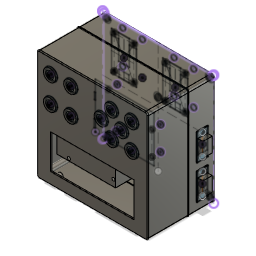
ArduinoController v4 (Autodesk Fusion 360 design; units mm, degrees)
Autodesk Fusion 360 part; units mm, degrees
sketch "Sketch1" plane through (0, 0, 0) normal (0, 0, 1) x (1, 0, 0) in component "RelayBoard"
  line L0 (22.5, -14.5) -> (-22.5, -14.5)
  line L1 (-22.5, -14.5) -> (-22.5, 14.5)
  line L2 (-22.5, 14.5) -> (22.5, 14.5)
  line L3 (22.5, 14.5) -> (22.5, -14.5)
  line L4 (22.5, -14.5) -> (-22.5, 14.5) construction
  line L5 (-22.5, -14.5) -> (22.5, 14.5) construction
  line L6 (19.5, -11.5) -> (-19.5, -11.5) construction
  line L7 (-19.5, -11.5) -> (-19.5, 11.5) construction
  line L8 (-19.5, 11.5) -> (19.5, 11.5) construction
  line L9 (19.5, 11.5) -> (19.5, -11.5) construction
  line L10 (19.5, -11.5) -> (-19.5, 11.5) construction
  line L11 (-19.5, -11.5) -> (19.5, 11.5) construction
  circle A0 centre (-19.5, 11.5) radius 1.75
  circle A1 centre (-19.5, 11.5) radius 1
  line L12 (0, 14.5) -> (0, -14.5) construction
  line L13 (-22.5, 0) -> (22.5, 0) construction
  circle A2 centre (19.5, 11.5) radius 1
  circle A3 centre (19.5, 11.5) radius 1.75
  circle A4 centre (19.5, -11.5) radius 1.75
  circle A5 centre (19.5, -11.5) radius 1
  circle A6 centre (-19.5, -11.5) radius 1
  circle A7 centre (-19.5, -11.5) radius 1.75
  line L14 (-22.5, 5.75) -> (-14.5, 5.75)
  line L15 (-14.5, 5.75) -> (-14.5, -5.75)
  line L16 (-14.5, -5.75) -> (-22.5, -5.75)
  line L17 (-22.5, -5.75) -> (-22.5, 5.75)
  line L18 (-22.5, 0) -> (-14.5, 0) construction
  line L19 (22.5, 6.15) -> (-6.5, 6.15)
  line L20 (-6.5, 6.15) -> (-6.5, -6.15)
  line L21 (-6.5, -6.15) -> (22.5, -6.15)
  line L22 (22.5, -6.15) -> (22.5, 6.15)
  line L23 (-6.5, 0) -> (22.5, 0) construction
  line L24 (16.1, 14.5) -> (4.6, 14.5)
  line L25 (4.6, 14.5) -> (4.6, 6.5)
  line L26 (4.6, 6.5) -> (16.1, 6.5)
  line L27 (16.1, 6.5) -> (16.1, 14.5)
  line L28 (4.6, -14.5) -> (4.6, -6.5)
  line L29 (4.6, -6.5) -> (16.1, -6.5)
  line L30 (16.1, -14.5) -> (4.6, -14.5)
  line L31 (16.1, -6.5) -> (16.1, -14.5)
  dimension "d1" = 45
  dimension "d2" = 29
  dimension "d3" = 39
  dimension "d4" = 23
  dimension "d5" = 3.5
  dimension "d6" = 2
  dimension "d7" = 11.5
  dimension "d8" = 29
  dimension "d9" = 12.3
  dimension "d10" = 8
  dimension "d11" = 11.5
  dimension "d12" = 8
  dimension "d13" = 6.4
  constraint horizontal L0
  constraint perpendicular L0 L1
  constraint parallel L0 L2
  constraint parallel L1 L3
  constraint coincident L4 origin
  constraint coincident L5 origin
  constraint horizontal L6
  constraint perpendicular L6 L7
  constraint parallel L6 L8
  constraint parallel L7 L9
  constraint coincident L10 origin
  constraint coincident L11 origin
  constraint coincident L7.end L8.start
  constraint concentric A0 A1
  constraint midpoint L2 L12.start
  constraint midpoint L0 L12.end
  constraint midpoint L1 L13.start
  constraint midpoint L3 L13.end
  constraint symmetric A0 L12 A3
  constraint symmetric A1 L12 A2
  constraint symmetric A0 L13 A7
  constraint symmetric A1 L13 A6
  constraint symmetric L13 A2 A5
  constraint symmetric L13 A3 A4
  constraint horizontal L14
  constraint vertical L15
  constraint horizontal L16
  constraint vertical L17
  constraint coincident L1 L14.start
  constraint midpoint L17 L13.start
  constraint midpoint L15 L18.end
  constraint collinear L13 L18
  constraint horizontal L19
  constraint vertical L20
  constraint horizontal L21
  constraint vertical L22
  constraint coincident L3 L19.start
  constraint midpoint L20 L23.start
  constraint midpoint L22 L13.end
  constraint collinear L13 L23
  constraint horizontal L24
  constraint vertical L25
  constraint horizontal L26
  constraint vertical L27
  constraint coincident L2 L24.start
  constraint symmetric L13 L24.start L30.start
  constraint symmetric L13 L24.end L28.start
  constraint symmetric L13 L25.end L28.end
  constraint symmetric L13 L26.end L29.end
  measures "d1" distance of L1.end L2.end
  measures "d2" distance of L0.end L1.end
  measures "d3" distance of L7.end L8.end
  measures "d4" distance of L6.end L7.end
  measures "d5" diameter of A0
  measures "d6" diameter of A1
  measures "d7" distance of L14.start L16.end
  measures "d8" distance of L19.start L19.end
  measures "d9" distance of L19.start L21.end
  measures "d10" distance of L15.end L16.end
  measures "d11" distance of L24.start L24.end
  measures "d12" distance of L24.start L26.end
  measures "d13" distance of L3 L27
extrude "Extrude1" add sketch "Sketch1" against normal blind 1.7 contours L0 L1 L2 L3 L14 L15 L16 L19 L20 L21 L25 L26 L27 L28 L29 L31 | L0 L28 L29 L30 L31 | L3 L19 L20 L21 L22 | L1 L14 L15 L16 L17 | L2 L24 L25 L26 L27 makes body 1 in component "RelayBoard"
extrude "Extrude2" add sketch "Sketch1" along normal blind 8.9 contours L0 L28 L29 L30 L31 | L1 L14 L15 L16 L17 | L2 L24 L25 L26 L27 bodies 1 in component "RelayBoard"
extrude "Extrude3" add sketch "Sketch1" along normal blind 20.7 contours L3 L19 L20 L21 L22 bodies 1 in component "RelayBoard"
fillet "Fillet1" radius 3 4 edges at (22.5, 14.5, -0.85) (22.5, -14.5, -0.85) (-22.5, 14.5, -0.85) (-22.5, -14.5, -0.85) on bodies 1 in component "RelayBoard"
sketch "Sketch1 (2)" plane through (0, 0, 0) normal (0, 0, 1) x (1, 0, 0) in component "BananaSocket"
  circle A0 centre (0, 0) radius 7.15
  circle A1 centre (0, 0) radius 5.95
  line L0 (-2.4985, 5.4) -> (2.4985, 5.4)
  line L1 (-2.4985, -5.4) -> (2.4985, -5.4)
  dimension "d22" = 14.3
  dimension "d23" = 11.9
  dimension "d24" = 10.8
  dimension "d25" = 5.4
  constraint coincident A0.centre A1.centre
  constraint concentric A0 A1
  constraint coincident A1 L0.start
  constraint coincident A1 L0.end
  constraint horizontal L0
  constraint coincident A1 L1.start
  constraint coincident A1 L1.end
  constraint parallel L0 L1
  measures "d22" diameter of A0
  measures "d23" diameter of A1
  measures "d24" distance of L0 L1
  measures "d25" distance of A0.centre L0
extrude "Extrude1'" add sketch "Sketch1 (2)" along normal blind 2 separate body contours A0 | A1 L0 L1 | A1 L0 | A1 L1 makes body 2 in component "BananaSocket"
extrude "Extrude2'" add sketch "Sketch1 (2)" against normal blind 21.5 contours A1 L0 L1 bodies 2 in component "BananaSocket"
sketch "Sketch2" plane through (0, 0, -21.5) normal (0, 0, -1) x (-1, 0, 0) in component "BananaSocket"
  arc A0 (2.4985, -5.4) -> (2.4985, 5.4) centre (0, 0) ccw
  line L0 (2.4985, 5.4) -> (-2.4985, 5.4)
  arc A1 (-2.4985, 5.4) -> (-2.4985, -5.4) centre (0, 0) ccw
  line L1 (-2.4985, -5.4) -> (2.4985, -5.4)
  line L2 (0.4, -3) -> (-0.4, -3)
  line L3 (-0.4, -3) -> (-0.4, 3)
  line L4 (-0.4, 3) -> (0.4, 3)
  line L5 (0.4, 3) -> (0.4, -3)
  line L6 (0.4, -3) -> (-0.4, 3) construction
  line L7 (-0.4, -3) -> (0.4, 3) construction
  dimension "d30" = 0.8
  dimension "d31" = 6
  constraint horizontal L2
  constraint perpendicular L2 L3
  constraint parallel L2 L4
  constraint parallel L3 L5
  constraint coincident L6 A0.centre
  constraint coincident L7 A0.centre
  measures "d30" distance of L3.end L4.end
  measures "d31" distance of L2.end L3.end
extrude "Extrude3'" add sketch "Sketch2" along normal blind 8.8 contours L2 L3 L4 L5 bodies 2 in component "BananaSocket"
sketch "Sketch3" plane through (0, 0, 2) normal (0, 0, 1) x (1, 0, 0) in component "BananaSocket"
  circle A0 centre (0, 0) radius 7.15
  circle A1 centre (0, 0) radius 2
  circle A2 centre (0, 0) radius 3
  circle A3 centre (0, 0) radius 4.45
  dimension "d34" = 4
  dimension "d35" = 6
  dimension "d36" = 8.9
  constraint concentric A0 A1
  constraint coincident A0.centre A1.centre
  constraint concentric A2 A3
  measures "d34" diameter of A1
  measures "d35" diameter of A2
  measures "d36" diameter of A3
extrude "Extrude4" cut sketch "Sketch3" against normal blind 20 contours A1 | A3 bodies 2 in component "BananaSocket"
sketch "Sketch1 (3)" plane through (0, 0, 0) normal (0, 1, 0) x (1, 0, 0) in component "LCD-20x4"
  line L0 (49, 30.1) -> (-49, 30.1)
  line L1 (-49, 30.1) -> (-49, -30.1)
  line L2 (-49, -30.1) -> (49, -30.1)
  line L3 (49, -30.1) -> (49, 30.1)
  line L4 (49, 30.1) -> (-49, -30.1) construction
  line L5 (-49, 30.1) -> (49, -30.1) construction
  line L6 (46.5, 27.625) -> (-46.5, 27.625) construction
  line L7 (-46.5, 27.625) -> (-46.5, -27.625) construction
  line L8 (-46.5, -27.625) -> (46.5, -27.625) construction
  line L9 (46.5, -27.625) -> (46.5, 27.625) construction
  line L10 (46.5, 27.625) -> (-46.5, -27.625) construction
  line L11 (-46.5, 27.625) -> (46.5, -27.625) construction
  circle A0 centre (-46.5, -27.625) radius 1.75
  circle A1 centre (-46.5, -27.625) radius 1
  line L12 (-49, 0) -> (49, 0) construction
  line L13 (0, -30.1) -> (0, 30.1) construction
  circle A2 centre (46.5, -27.625) radius 1
  circle A3 centre (46.5, -27.625) radius 1.75
  circle A4 centre (-46.5, 27.625) radius 1
  circle A5 centre (-46.5, 27.625) radius 1.75
  circle A6 centre (46.5, 27.625) radius 1.75
  circle A7 centre (46.5, 27.625) radius 1
  line L14 (48.6, 19.9) -> (-48.6, 19.9)
  line L15 (-48.6, 19.9) -> (-48.6, -19.9)
  line L16 (-48.6, -19.9) -> (48.6, -19.9)
  line L17 (48.6, -19.9) -> (48.6, 19.9)
  line L18 (48.6, 19.9) -> (-48.6, -19.9) construction
  line L19 (-48.6, 19.9) -> (48.6, -19.9) construction
  line L20 (40, 30.1) -> (0, 30.1)
  line L21 (0, 30.1) -> (0, 27.1)
  line L22 (0, 27.1) -> (40, 27.1)
  line L23 (40, 27.1) -> (40, 30.1)
  dimension "d39" = 98
  dimension "d40" = 60.2
  dimension "d41" = 93
  dimension "d42" = 55.25
  dimension "d43" = 3.5
  dimension "d44" = 2
  dimension "d45" = 97.2
  dimension "d46" = 39.8
  dimension "d51" = 40
  dimension "d52" = 3
  dimension "d53" = 9
  constraint horizontal L0
  constraint perpendicular L0 L1
  constraint parallel L0 L2
  constraint parallel L1 L3
  constraint coincident L4 origin
  constraint coincident L5 origin
  constraint horizontal L6
  constraint perpendicular L6 L7
  constraint parallel L6 L8
  constraint parallel L7 L9
  constraint coincident L10 origin
  constraint coincident L11 origin
  constraint coincident L7.end L8.start
  constraint concentric A0 A1
  constraint midpoint L1 L12.start
  constraint midpoint L3 L12.end
  constraint midpoint L2 L13.start
  constraint midpoint L0 L13.end
  constraint symmetric A0 L13 A3
  constraint symmetric A1 L13 A2
  constraint symmetric A0 L12 A5
  constraint symmetric A1 L12 A4
  constraint symmetric L12 A2 A7
  constraint symmetric L12 A3 A6
  constraint horizontal L14
  constraint perpendicular L14 L15
  constraint parallel L14 L16
  constraint parallel L15 L17
  constraint coincident L18 origin
  constraint coincident L19 origin
  constraint horizontal L20
  constraint vertical L21
  constraint horizontal L22
  constraint vertical L23
  constraint coincident L0 L20.start
  measures "d39" distance of L1.end L2.end
  measures "d40" distance of L0.end L1.end
  measures "d41" distance of L7.end L8.end
  measures "d42" distance of L6.end L7.end
  measures "d43" diameter of A0
  measures "d44" diameter of A1
  measures "d45" distance of L15.end L16.end
  measures "d46" distance of L14.end L15.end
  measures "d51" distance of L20.start L13.end
  measures "d52" distance of L20.start L22.end
  measures "d53" distance of L3 L23
extrude "Extrude1''" add sketch "Sketch1 (3)" against normal blind 9.6 separate body contours L14 L15 L16 L17 makes body 3 in component "LCD-20x4"
extrude "Extrude2''" add sketch "Sketch1 (3)" along normal blind 1.7 contours L0 L1 L2 L3 L21 L22 L23 | L0 L20 L21 L22 L23 | L14 L15 L16 L17 bodies 3 in component "LCD-20x4"
extrude "Extrude3''" add sketch "Sketch1 (3)" against normal blind 4 contours L0 L20 L21 L22 L23 bodies 3 in component "LCD-20x4"
sketch "Sketch2 (2)" plane through (0, 1.7, 0) normal (0, 1, 0) x (-1, 0, 0) in component "LCD-20x4"
  circle A0 centre (-46.5, -27.625) radius 1.75
  circle A1 centre (46.5, -27.625) radius 1.75
  circle A2 centre (-46.5, 27.625) radius 1.75
  circle A3 centre (46.5, 27.625) radius 1.75
  line L0 (-49, 30.1) -> (-49, -30.1)
  line L1 (-49, -30.1) -> (49, -30.1)
  line L2 (49, -30.1) -> (49, 30.1)
  line L3 (49, 30.1) -> (-49, 30.1)
  line L4 (-49, -30.1) -> (7, -30.1)
  line L5 (7, -30.1) -> (7, -10.1)
  line L6 (7, -10.1) -> (-49, -10.1)
  line L7 (-49, -10.1) -> (-49, -30.1)
  line L8 (-49, -30.1) -> (-41, -30.1)
  line L9 (-41, -30.1) -> (-41, -24.1)
  line L10 (-41, -24.1) -> (-49, -24.1)
  line L11 (-49, -24.1) -> (-49, -30.1)
  line L12 (-49, -24.1) -> (-61, -24.1)
  line L13 (-61, -24.1) -> (-61, -14.1)
  line L14 (-61, -14.1) -> (-49, -14.1)
  line L15 (-49, -14.1) -> (-49, -24.1)
  dimension "d56" = 56
  dimension "d57" = 20
  dimension "d58" = 8
  dimension "d59" = 6
  dimension "d60" = 12
  dimension "d61" = 10
  constraint horizontal L4
  constraint vertical L5
  constraint horizontal L6
  constraint vertical L7
  constraint coincident L0.end L1.start
  constraint horizontal L8
  constraint vertical L9
  constraint horizontal L10
  constraint vertical L11
  constraint horizontal L12
  constraint vertical L13
  constraint horizontal L14
  constraint vertical L15
  measures "d56" distance of L0.end L4.end
  measures "d57" distance of L0.end L6.end
  measures "d58" distance of L0.end L8.end
  measures "d59" distance of L0.end L10.end
  measures "d60" distance of L10.end L12.end
  measures "d61" distance of L10.end L14.end
extrude "Extrude4'" add sketch "Sketch2 (2)" along normal blind 10 contours L0 L1 L4 L5 L6 L7 L9 L10 L15 | L0 L7 L12 L13 L14 L15 bodies 3 in component "LCD-20x4"
sketch "Sketch1 (4)" plane through (0, 0, 0) normal (0, 0, 1) x (1, 0, 0) in component "db9"
  line L0 (15.4, -6.25) -> (-15.4, -6.25)
  line L1 (-15.4, -6.25) -> (-15.4, 6.25)
  line L2 (-15.4, 6.25) -> (15.4, 6.25)
  line L3 (15.4, 6.25) -> (15.4, -6.25)
  line L4 (15.4, -6.25) -> (-15.4, 6.25) construction
  line L5 (-15.4, -6.25) -> (15.4, 6.25) construction
  line L6 (-12.5, 0) -> (12.5, 0) construction
  circle A0 centre (-12.5, 0) radius 1.75
  circle A1 centre (-12.5, 0) radius 1
  circle A2 centre (12.5, 0) radius 1.75
  circle A3 centre (12.5, 0) radius 1
  line L7 (8.5, -5.5) -> (-8.5, -5.5)
  line L8 (-8.5, -5.5) -> (-8.5, 5.5)
  line L9 (-8.5, 5.5) -> (8.5, 5.5)
  line L10 (8.5, 5.5) -> (8.5, -5.5)
  line L11 (8.5, -5.5) -> (-8.5, 5.5) construction
  line L12 (-8.5, -5.5) -> (8.5, 5.5) construction
  dimension "d64" = 30.8
  dimension "d65" = 12.5
  dimension "d66" = 25
  dimension "d67" = 12.5
  dimension "d68" = 3.5
  dimension "d69" = 2
  dimension "d70" = 3.5
  dimension "d71" = 2
  dimension "d72" = 17
  dimension "d73" = 11
  constraint horizontal L0
  constraint perpendicular L0 L1
  constraint parallel L0 L2
  constraint parallel L1 L3
  constraint coincident L4 origin
  constraint coincident L5 origin
  constraint horizontal L6
  constraint coincident L6.start A0.centre
  constraint concentric A0 A1
  constraint coincident L6.end A2.centre
  constraint concentric A2 A3
  constraint horizontal L7
  constraint perpendicular L7 L8
  constraint parallel L7 L9
  constraint parallel L8 L10
  constraint coincident L11 origin
  constraint coincident L12 origin
  measures "d64" distance of L1.end L2.end
  measures "d65" distance of L0.end L1.end
  measures "d66" distance of L6.start L6.end
  measures "d67" distance of origin L6.end
  measures "d68" diameter of A0
  measures "d69" diameter of A1
  measures "d70" diameter of A2
  measures "d71" diameter of A3
  measures "d72" distance of L8.end L9.end
  measures "d73" distance of L7.end L8.end
extrude "Extrude1'''" add sketch "Sketch1 (4)" against normal blind 1 separate body contours L0 L1 L2 L3 | L7 L8 L9 L10 makes body 4 in component "db9"
extrude "Extrude2'''" add sketch "Sketch1 (4)" along normal blind 6 contours L7 L8 L9 L10 bodies 4 in component "db9"
sketch "Sketch2 (3)" plane through (0, 0, -1) normal (0, 0, -1) x (-1, 0, 0) in component "db9"
  circle A0 centre (-12.5, 0) radius 1.75
  circle A1 centre (12.5, 0) radius 1.75
  line L0 (15.4, 6.25) -> (-15.4, 6.25)
  line L1 (-15.4, 6.25) -> (-15.4, -6.25)
  line L2 (-15.4, -6.25) -> (15.4, -6.25)
  line L3 (15.4, -6.25) -> (15.4, 6.25)
  line L4 (9.65, -5.5) -> (-9.65, -5.5)
  line L5 (-9.65, -5.5) -> (-9.65, 5.5)
  line L6 (-9.65, 5.5) -> (9.65, 5.5)
  line L7 (9.65, 5.5) -> (9.65, -5.5)
  line L8 (9.65, -5.5) -> (-9.65, 5.5) construction
  line L9 (-9.65, -5.5) -> (9.65, 5.5) construction
  dimension "d78" = 19.3
  dimension "d79" = 11
  constraint horizontal L4
  constraint perpendicular L4 L5
  constraint parallel L4 L6
  constraint parallel L5 L7
  constraint coincident L8 origin
  constraint coincident L9 origin
  measures "d78" distance of L5.end L6.end
  measures "d79" distance of L4.end L5.end
extrude "Extrude3'''" add sketch "Sketch2 (3)" along normal blind 13 contours L4 L5 L6 L7 bodies 4 in component "db9"
sketch "Sketch1 (5)" plane through (0, 0, 0) normal (0, 0, 1) x (1, 0, 0) in component "ArduinoWithCNCshield"
  line L0 (0, 0) -> (68.6, 0)
  line L1 (68.6, 0) -> (68.6, 53.3)
  line L2 (68.6, 53.3) -> (0, 53.3)
  line L3 (0, 53.3) -> (0, 0)
  circle A0 centre (14, 2.5) radius 1.75
  circle A1 centre (14, 2.5) radius 1
  circle A2 centre (66.1, 7.6) radius 1.75
  circle A3 centre (15.3, 50.7) radius 1.75
  circle A4 centre (66.1, 35.5) radius 1.75
  line L4 (66.1, 35.5) -> (66.1, 7.6) construction
  line L5 (0, 3.7) -> (-1.5, 3.7)
  line L6 (-1.5, 3.7) -> (-1.5, 12.6)
  line L7 (-1.5, 12.6) -> (0, 12.6)
  line L8 (0, 12.6) -> (0, 3.7)
  line L9 (0, 39.9) -> (-1, 39.9)
  line L10 (-1, 39.9) -> (-1, 32.4)
  line L11 (-1, 32.4) -> (0, 32.4)
  line L12 (0, 32.4) -> (0, 39.9)
  dimension "d82" = 68.6
  dimension "d83" = 53.3
  dimension "d84" = 3.5
  dimension "d85" = 2
  dimension "d86" = 2.5
  dimension "d87" = 14
  dimension "d88" = 3.5
  dimension "d89" = 3.5
  dimension "d90" = 1.3
  dimension "d91" = 3.5
  dimension "d92" = 50.8
  dimension "d93" = 5.1
  dimension "d94" = 27.9
  dimension "d95" = 15.2
  dimension "d96" = 1.5
  dimension "d97" = 8.9
  dimension "d98" = 3.7
  dimension "d99" = 1
  dimension "d100" = 7.5
  dimension "d101" = 13.4
  constraint horizontal L0
  constraint vertical L1
  constraint horizontal L2
  constraint vertical L3
  constraint coincident L0.start L3.end
  constraint concentric A0 A1
  constraint coincident A4.centre L4.start
  constraint coincident A2.centre L4.end
  constraint vertical L4
  constraint horizontal L5
  constraint vertical L6
  constraint horizontal L7
  constraint vertical L8
  constraint coincident L3 L5.start
  constraint horizontal L9
  constraint vertical L10
  constraint horizontal L11
  constraint vertical L12
  constraint coincident L3 L9.start
  measures "d82" distance of L0.start L0.end
  measures "d83" distance of L0.start L2.end
  measures "d84" diameter of A0
  measures "d85" diameter of A1
  measures "d86" distance of L0 A0.centre
  measures "d87" distance of L3 A0.centre
  measures "d88" diameter of A2
  measures "d89" diameter of A3
  measures "d90" horizontal distance of A0.centre A3.centre
  measures "d91" diameter of A4
  measures "d92" horizontal distance of A3.centre A4.centre
  measures "d93" vertical distance of A0.centre A2.centre
  measures "d94" distance of A4.centre A2.centre
  measures "d95" vertical distance of A3.centre A4.centre
  measures "d96" distance of L5.start L5.end
  measures "d97" distance of L5.start L7.end
  measures "d98" distance of L0 L5
  measures "d99" distance of L9.start L9.end
  measures "d100" distance of L9.start L11.end
  measures "d101" distance of L2 L9
extrude "Extrude1''''" add sketch "Sketch1 (5)" along normal blind 45 separate body contours L0 L1 L2 L3 L8 L12 makes body 5 in component "ArduinoWithCNCshield"
extrude "Extrude2''''" add sketch "Sketch1 (5)" along normal blind 11 contours L3 L5 L6 L7 L8 bodies 5 in component "ArduinoWithCNCshield"
extrude "Extrude3''''" add sketch "Sketch1 (5)" along normal blind 4 contours L3 L9 L10 L11 L12 bodies 5 in component "ArduinoWithCNCshield"
extrude "Extrude4''" add sketch "Sketch1 (5)" against normal blind 1.7 contours L0 L1 L2 L3 L8 L12 bodies 5 in component "ArduinoWithCNCshield"
sketch "Sketch1 (6)" plane through (0, 0, 0) normal (0, 0, 1) x (1, 0, 0)
  line L0 (65, -65) -> (-65, -65)
  line L1 (-65, -65) -> (-65, 65)
  line L2 (-65, 65) -> (65, 65)
  line L3 (65, 65) -> (65, -65)
  line L4 (65, -65) -> (-65, 65) construction
  line L5 (-65, -65) -> (65, 65) construction
  line L6 (63.5, -63.5) -> (-63.5, -63.5)
  line L7 (-63.5, -63.5) -> (-63.5, 63.5)
  line L8 (-63.5, 63.5) -> (63.5, 63.5)
  line L9 (63.5, 63.5) -> (63.5, -63.5)
  line L10 (63.5, -63.5) -> (-63.5, 63.5) construction
  line L11 (-63.5, -63.5) -> (63.5, 63.5) construction
  dimension "d110" = 130
  dimension "d111" = 130
  dimension "d112" = 1.5
  dimension "d113" = 1.5
  constraint horizontal L0
  constraint perpendicular L0 L1
  constraint parallel L0 L2
  constraint parallel L1 L3
  constraint coincident L4 origin
  constraint coincident L5 origin
  constraint horizontal L6
  constraint perpendicular L6 L7
  constraint parallel L6 L8
  constraint parallel L7 L9
  constraint coincident L10 origin
  constraint coincident L11 origin
  measures "d110" distance of L1.end L2.end
  measures "d111" distance of L0.end L1.end
  measures "d112" distance of L2 L8
  measures "d113" distance of L1 L7
extrude "Extrude1'''''" add sketch "Sketch1 (6)" against normal blind 1.5 separate body contours L0 L1 L2 L3 | L6 L7 L8 L9 makes body 6
extrude "Extrude2'''''" add sketch "Sketch1 (6)" along normal blind 30 bodies 6
sketch "Sketch4" plane through (0, -11, 77.1) normal (0, 0, 1) x (1, 0, 0)
  line L0 (-48.6, -0.1) -> (-48.6, -39.9)
  line L1 (-48.6, -39.9) -> (48.6, -39.9)
  line L2 (48.6, -39.9) -> (48.6, -0.1)
  line L3 (48.6, -0.1) -> (-48.6, -0.1)
  line L4 (65, 76) -> (65, -54)
  line L5 (65, -54) -> (-65, -54)
  line L6 (-65, -54) -> (-65, 76)
  line L7 (-65, 76) -> (65, 76)
  line L8 (-48.85, -40.15) -> (48.85, -40.15)
  line L9 (48.85, -40.15) -> (48.85, 0.15)
  line L10 (48.85, 0.15) -> (-48.85, 0.15)
  line L11 (-48.85, 0.15) -> (-48.85, -40.15)
  circle A0 centre (46.5, 7.625) radius 1
  circle A1 centre (-46.5, 7.625) radius 1
  circle A2 centre (-46.5, -47.625) radius 1
  circle A3 centre (46.5, -47.625) radius 1
  circle A4 centre (-46.5, 7.625) radius 3
  circle A5 centre (-46.5, -47.625) radius 3
  circle A6 centre (46.5, -47.625) radius 3
  circle A7 centre (46.5, 7.625) radius 3
  line L12 (-18, 29) -> (-48, 29) construction
  line L13 (-48, 29) -> (-48, 59) construction
  line L14 (-48, 59) -> (-18, 59) construction
  line L15 (-18, 59) -> (-18, 29) construction
  line L16 (-18, 29) -> (-48, 59) construction
  line L17 (-48, 29) -> (-18, 59) construction
  line L18 (-33, 44) -> (33, 44) construction
  line L19 (51, 26) -> (15, 26) construction
  line L20 (15, 26) -> (15, 62) construction
  line L21 (15, 62) -> (51, 62) construction
  line L22 (51, 62) -> (51, 26) construction
  line L23 (51, 26) -> (15, 62) construction
  line L24 (15, 26) -> (51, 62) construction
  line L25 (15, 62) -> (-3, 44) construction
  circle A8 centre (-48, 59) radius 6.15
  line L26 (-50.7518, 64.5) -> (-45.2482, 64.5)
  line L27 (-50.7518, 53.5) -> (-45.2482, 53.5)
  circle A9 centre (-24.25, 59) radius 6.15
  line L28 (-27.0018, 64.5) -> (-21.4982, 64.5)
  line L29 (-27.0018, 53.5) -> (-21.4982, 53.5)
  circle A10 centre (23.25, 59) radius 6.15
  line L30 (20.4982, 64.5) -> (26.0018, 64.5)
  line L31 (20.4982, 53.5) -> (26.0018, 53.5)
  circle A11 centre (47, 59) radius 6.15
  line L32 (44.2482, 64.5) -> (49.7518, 64.5)
  line L33 (44.2482, 53.5) -> (49.7518, 53.5)
  circle A12 centre (11.375, 44) radius 6.15
  line L34 (8.6232, 49.5) -> (14.1268, 49.5)
  line L35 (8.6232, 38.5) -> (14.1268, 38.5)
  circle A13 centre (35.125, 44) radius 6.15
  line L36 (32.3732, 49.5) -> (37.8768, 49.5)
  line L37 (32.3732, 38.5) -> (37.8768, 38.5)
  circle A14 centre (-48, 29) radius 6.15
  line L38 (-50.7518, 34.5) -> (-45.2482, 34.5)
  line L39 (-50.7518, 23.5) -> (-45.2482, 23.5)
  circle A15 centre (-24.25, 29) radius 6.15
  line L40 (-27.0018, 34.5) -> (-21.4982, 34.5)
  line L41 (-27.0018, 23.5) -> (-21.4982, 23.5)
  circle A16 centre (23.25, 29) radius 6.15
  line L42 (20.4982, 34.5) -> (26.0018, 34.5)
  line L43 (20.4982, 23.5) -> (26.0018, 23.5)
  circle A17 centre (47, 29) radius 6.15
  line L44 (44.2482, 34.5) -> (49.7518, 34.5)
  line L45 (44.2482, 23.5) -> (49.7518, 23.5)
  line L46 (63.5, -52.5) -> (-63.5, -52.5)
  line L47 (-63.5, -52.5) -> (-63.5, 74.5)
  line L48 (-63.5, 74.5) -> (63.5, 74.5)
  line L49 (63.5, 74.5) -> (63.5, -52.5)
  circle A18 centre (-60.25, 71.25) radius 3.25
  circle A19 centre (-60.25, 71.25) radius 1
  line L50 (0, 76) -> (0, -54) construction
  line L51 (-65, 11) -> (65, 11) construction
  circle A20 centre (60.25, 71.25) radius 3.25
  circle A21 centre (60.25, 71.25) radius 1
  circle A22 centre (-60.25, -49.25) radius 1
  circle A23 centre (-60.25, -49.25) radius 3.25
  circle A24 centre (60.25, -49.25) radius 3.25
  circle A25 centre (60.25, -49.25) radius 1
  circle A26 centre (0, 21) radius 1
  circle A27 centre (0, 21) radius 3.25
  point P0 (-33, 44)
  point P1 (33, 44)
  point P2 (0, 11)
  dimension "d134" = 0.25
  dimension "d137" = 6
  dimension "d138" = 6
  dimension "d139" = 6
  dimension "d140" = 6
  dimension "d143" = 30
  dimension "d144" = 32
  dimension "d145" = 32
  dimension "d146" = 36
  dimension "d147" = 36
  dimension "d148" = 30
  dimension "d150" = 66
  dimension "d151" = 12.3
  dimension "d152" = 11
  dimension "d153" = 5.5
  dimension "d156" = 95
  dimension "d157" = -30
  dimension "d200" = 1.5
  dimension "d201" = 1.5
  dimension "d202" = 1.5
  dimension "d203" = 1.5
  dimension "d211" = 6.5
  dimension "d212" = 2
  dimension "d218" = 2
  dimension "d219" = 6.5
  dimension "d220" = 10
  constraint concentric A1 A4
  constraint concentric A2 A5
  constraint concentric A3 A6
  constraint concentric A0 A7
  constraint horizontal L12
  constraint perpendicular L12 L13
  constraint parallel L12 L14
  constraint parallel L13 L15
  constraint coincident L16 P0
  constraint coincident L17 P0
  constraint coincident P0 L18.start
  constraint perpendicular L15 L18
  constraint horizontal L19
  constraint perpendicular L19 L20
  constraint parallel L19 L21
  constraint parallel L20 L22
  constraint coincident L23 P1
  constraint coincident L24 P1
  constraint coincident P1 L18.end
  constraint coincident L18 L25.end
  constraint perpendicular L23 L25
  constraint coincident L13.end L14.start
  constraint coincident A8 L26.start
  constraint coincident A8 L26.end
  constraint horizontal L26
  constraint coincident A8 L27.start
  constraint coincident A8 L27.end
  constraint perpendicular L13 L27
  constraint horizontal L46
  constraint vertical L47
  constraint horizontal L48
  constraint vertical L49
  constraint tangent L48 A18
  constraint tangent L47 A18
  constraint concentric A18 A19
  constraint midpoint L7 L50.start
  constraint midpoint L5 L50.end
  constraint midpoint L6 L51.start
  constraint midpoint L4 L51.end
  constraint symmetric A18 L50 A20
  constraint symmetric A19 L50 A21
  constraint symmetric A18 L51 A23
  constraint symmetric A19 L51 A22
  constraint symmetric L51 A20 A24
  constraint symmetric L51 A21 A25
  constraint coincident L50 A26.centre
  constraint concentric A26 A27
  measures "d137" diameter of A4
  measures "d138" diameter of A5
  measures "d139" diameter of A6
  measures "d140" diameter of A7
  measures "d143" distance of L12.end L13.end
  measures "d144" distance of L7 P0
  measures "d145" distance of L6 P0
  measures "d146" distance of L20.end L21.end
  measures "d147" distance of L19.end L20.end
  measures "d148" distance of L12.start L12.end
  measures "d150" distance of P0 P1
  measures "d151" diameter of A8
  measures "d152" distance of L26 L27
  measures "d153" distance of L13.end L26
  measures "d200" distance of L4.end L49
  measures "d201" distance of L4.end L46
  measures "d202" distance of L5.end L47
  measures "d203" distance of L4.start L48
  measures "d211" diameter of A18
  measures "d212" diameter of A19
  measures "d218" diameter of A26
  measures "d219" diameter of A27
  measures "d220" distance of A26.centre P2
extrude "Extrude3'''''" add sketch "Sketch4" against normal blind 1.5 separate body contours L4 L5 L6 L7 | A0 | A1 | A2 | A3 | A4 | A5 | A6 | A7 | A8 L26 L27 | A8 L26 | A8 L27 | A9 L28 L29 | A9 L28 | A9 L29 | A10 L30 L31 | A10 L30 | A10 L31 | A11 L32 L33 | A11 L32 | A11 L33 | A12 L34 L35 | A12 L34 | A12 L35 | A13 L36 L37 | A13 L36 | A13 L37 | A14 L38 L39 | A14 L38 | A14 L39 | A15 L40 L41 | A15 L40 | A15 L41 | A16 L42 L43 | A16 L42 | A16 L43 | A17 L44 L45 | A17 L44 | A17 L45 | L46 L49 A24 | L46 L47 L48 L49 A18 A20 A23 A24 | A24 | L46 L47 A23 | A23 | L48 L49 A20 | A20 | L47 L48 A18 | A18 | A19 | A21 | A22 | A25 | A26 | A27 makes body 7
extrude "Extrude4'''" add sketch "Sketch4" against normal blind 9.5 contours A4 | A5 | A6 | A7 bodies 7
extrude "Extrude5" cut sketch "Sketch4" against normal blind 1.5 contours A8 L26 L27 | A9 L28 L29 | A10 L30 L31 | A11 L32 L33 | A12 L34 L35 | A13 L36 L37 | A14 L38 L39 | A15 L40 L41 | A16 L42 L43 | A17 L44 L45 bodies 7
extrude "Extrude6" add sketch "Sketch4" against normal blind 47 contours L4 L5 L6 L7 bodies 7
sketch "Sketch5" plane through (0, 0, 0) normal (0, 0, 1) x (1, 0, 0)
  circle A0 centre (-60.25, 60.25) radius 3.25
  line L0 (-63.5, 63.5) -> (63.5, 63.5)
  circle A1 centre (-60.25, 60.25) radius 4.75
  line L1 (-65, 65) -> (65, 65)
  line L2 (0, 65) -> (0, -65) construction
  line L3 (-65, 0) -> (65, 0) construction
  line L4 (-65, -65) -> (-65, 65) construction
  line L5 (65, 65) -> (65, -65) construction
  circle A2 centre (60.25, 60.25) radius 3.25
  circle A3 centre (60.25, 60.25) radius 4.75
  circle A4 centre (60.25, -60.25) radius 4.75
  circle A5 centre (60.25, -60.25) radius 3.25
  circle A6 centre (-60.25, -60.25) radius 3.25
  circle A7 centre (-60.25, -60.25) radius 4.75
  line L6 (-63.5, -63.5) -> (-63.5, 63.5)
  circle A8 centre (0, 10) radius 3.25
  circle A9 centre (0, 10) radius 4.75
  circle A10 centre (-41.5, 20.5) radius 1
  circle A11 centre (-18.5, 59.5) radius 1
  circle A12 centre (-41.5, 59.5) radius 1
  circle A13 centre (18.5, 59.5) radius 1
  circle A14 centre (41.5, 59.5) radius 1
  circle A15 centre (41.5, 20.5) radius 1
  circle A16 centre (18.5, 20.5) radius 1
  circle A17 centre (-48, -0.95) radius 1.75
  circle A18 centre (-49.3, -49.15) radius 1.75
  circle A19 centre (2.8, -44.05) radius 1.75
  circle A20 centre (2.8, -16.15) radius 1.75
  circle A21 centre (-41.5, 59.5) radius 3.25
  circle A22 centre (-18.5, 59.5) radius 3.25
  circle A23 centre (-41.5, 20.5) radius 3.25
  circle A24 centre (-18.5, 20.5) radius 3.25
  circle A25 centre (18.5, 59.5) radius 3.25
  circle A26 centre (41.5, 59.5) radius 3.25
  circle A27 centre (18.5, 20.5) radius 3.25
  circle A28 centre (41.5, 20.5) radius 3.25
  circle A29 centre (-48, -0.95) radius 3.25
  circle A30 centre (2.8, -16.15) radius 3.25
  circle A31 centre (2.8, -44.05) radius 3.25
  circle A32 centre (-49.3, -49.15) radius 3.25
  circle A33 centre (-49.3, -49.15) radius 1
  circle A34 centre (-48, -0.95) radius 1
  circle A35 centre (2.8, -16.15) radius 1
  circle A36 centre (2.8, -44.05) radius 1
  circle A37 centre (-18.5, 20.5) radius 1
  point P0 (-18.5, 20.5)
  dimension "d206" = 6.5
  dimension "d215" = 6.5
  dimension "d216" = 9.5
  dimension "d217" = 10
  dimension "d226" = 6.5
  dimension "d227" = 6.5
  dimension "d228" = 6.5
  dimension "d229" = 6.5
  dimension "d230" = 6.5
  dimension "d231" = 6.5
  dimension "d232" = 6.5
  dimension "d233" = 6.5
  dimension "d234" = 6.5
  dimension "d235" = 6.5
  dimension "d236" = 6.5
  dimension "d237" = 6.5
  dimension "d238" = 2
  dimension "d239" = 2
  dimension "d240" = 2
  dimension "d241" = 2
  dimension "d242" = 2
  constraint tangent A0 L0
  constraint concentric A0 A1
  constraint tangent A1 L1
  constraint midpoint L1 L2.start
  constraint perpendicular L0 L2
  constraint midpoint L3.start L4
  constraint midpoint L3.end L5
  constraint symmetric A0 L2 A2
  constraint symmetric A1 L2 A3
  constraint symmetric A0 L3 A6
  constraint symmetric A1 L3 A7
  constraint symmetric L3 A2 A5
  constraint symmetric L3 A3 A4
  constraint tangent A0 L6
  constraint coincident L2 A8.centre
  constraint concentric A8 A9
  constraint concentric A12 A21
  constraint concentric A11 A22
  constraint concentric A10 A23
  constraint coincident P0 A24.centre
  constraint concentric A13 A25
  constraint concentric A14 A26
  constraint concentric A16 A27
  constraint concentric A15 A28
  constraint concentric A17 A29
  constraint concentric A20 A30
  constraint concentric A19 A31
  constraint concentric A18 A32
  constraint concentric A32 A33
  constraint concentric A29 A34
  constraint concentric A30 A35
  constraint concentric A19 A36
  measures "d206" diameter of A0
  measures "d215" diameter of A8
  measures "d216" diameter of A9
  measures "d217" distance of origin A8.centre
  measures "d226" diameter of A21
  measures "d227" diameter of A22
  measures "d228" diameter of A23
  measures "d229" diameter of A24
  measures "d230" diameter of A25
  measures "d231" diameter of A26
  measures "d232" diameter of A27
  measures "d233" diameter of A28
  measures "d234" diameter of A29
  measures "d235" diameter of A30
  measures "d236" diameter of A31
  measures "d237" diameter of A32
  measures "d238" diameter of A33
  measures "d239" diameter of A34
  measures "d240" diameter of A35
  measures "d241" diameter of A36
  measures "d242" diameter of A37
extrude "Extrude7" add sketch "Sketch5" along normal blind 30 contours A0 L0 A1 L6 | A0 L0 L6 | L0 A1 L6 | A3 | A4 | A7 | A9 bodies 6
extrude "Extrude8" cut 5 faces at (58.3846, 59.3517, 0) (-62.1154, 59.3517, 0) (-62.1154, -61.1483, 0) (60.9536, -61.1882, 0) (0.3002, 8.7931, 0) along direction (0, 0, -1) blind 1.5 on bodies 6 bodies 6
extrude "Extrude9" add sketch "Sketch4" against normal blind 47 contours L46 L49 A24 | A24 | L46 L47 A23 | A23 | L48 L49 A20 | A20 | L47 L48 A18 | A18 | A27 bodies 7
sketch "Sketch6" plane through (0, 0, 30) normal (0, 0, 1) x (1, 0, 0)
  line L0 (56.7859, -63.5) -> (-56.7859, -63.5)
  arc A0 (-56.7859, -63.5) -> (-63.5, -56.7859) centre (-60.25, -60.25) ccw
  line L1 (-63.5, -56.7859) -> (-63.5, 56.7859)
  arc A1 (-63.5, 56.7859) -> (-56.7859, 63.5) centre (-60.25, 60.25) ccw
  line L2 (-56.7859, 63.5) -> (56.7859, 63.5)
  arc A2 (56.7859, 63.5) -> (63.5, 56.7859) centre (60.25, 60.25) ccw
  line L3 (63.5, 56.7859) -> (63.5, -56.7859)
  arc A3 (63.5, -56.7859) -> (56.7859, -63.5) centre (60.25, -60.25) ccw
  circle A4 centre (60.25, -60.25) radius 3.25
  circle A5 centre (60.25, 60.25) radius 3.25
  circle A6 centre (-60.25, 60.25) radius 3.25
  circle A7 centre (-60.25, -60.25) radius 3.25
  line L4 (-65, -65) -> (65, -65)
  line L5 (65, -65) -> (65, 65)
  line L6 (65, 65) -> (-65, 65)
  line L7 (-65, 65) -> (-65, -65)
  circle A8 centre (60.25, -60.25) radius 1.75
  circle A9 centre (60.25, -60.25) radius 3.25
  circle A10 centre (-60.25, -60.25) radius 3.25
  circle A11 centre (0, 10) radius 3.25
  circle A12 centre (60.25, 60.25) radius 3.25
  circle A13 centre (-60.25, 60.25) radius 3.25
  circle A14 centre (60.25, 60.25) radius 1.75
  circle A15 centre (-60.25, 60.25) radius 1.75
  circle A16 centre (0, 10) radius 1.75
  circle A17 centre (-60.25, -60.25) radius 1.75
  dimension "d221" = 3.5
  dimension "d222" = 3.5
  dimension "d223" = 3.5
  dimension "d224" = 3.5
  dimension "d225" = 3.5
  constraint concentric A3 A8
  constraint concentric A12 A14
  constraint concentric A13 A15
  constraint concentric A11 A16
  constraint concentric A0 A17
  measures "d221" diameter of A8
  measures "d222" diameter of A14
  measures "d223" diameter of A15
  measures "d224" diameter of A16
  measures "d225" diameter of A17
extrude "Extrude10" add sketch "Sketch5" along normal blind 10 contours A17 | A18 | A19 | A20 | A21 | A22 | A23 | A24 | A25 | A26 | A27 | A28 | A29 | A30 | A31 | A32 bodies 6
sketch "Sketch7" plane through (-65, 0, 0) normal (-1, 0, 0) x (0, 0, 1)
  line L0 (30, 65) -> (-1.5, 65)
  line L1 (-1.5, 65) -> (-1.5, -65)
  line L2 (-1.5, -65) -> (30, -65)
  line L3 (30, -65) -> (30, 65)
  line L4 (10.2, -11.75) -> (10.2, -19.25)
  line L5 (10.2, -19.25) -> (14.2, -19.25)
  line L6 (14.2, -19.25) -> (14.2, -11.75)
  line L7 (14.2, -11.75) -> (10.2, -11.75)
  line L8 (10.2, -39.05) -> (10.2, -47.95)
  line L9 (10.2, -47.95) -> (21.2, -47.95)
  line L10 (21.2, -47.95) -> (21.2, -39.05)
  line L11 (21.2, -39.05) -> (10.2, -39.05)
  line L12 (9.7, -38.55) -> (21.7, -38.55)
  line L13 (21.7, -38.55) -> (21.7, -48.45)
  line L14 (21.7, -48.45) -> (9.7, -48.45)
  line L15 (9.7, -48.45) -> (9.7, -38.55)
  line L16 (10.2, -47.95) -> (10.2, -39.05)
  line L17 (7.7, -9.25) -> (16.7, -9.25)
  line L18 (16.7, -9.25) -> (16.7, -21.75)
  line L19 (16.7, -21.75) -> (7.7, -21.75)
  line L20 (7.7, -21.75) -> (7.7, -9.25)
  line L21 (10.2, -11.75) -> (10.2, -19.25)
  dimension "d245" = 0.5
  dimension "d246" = 0.5
  dimension "d247" = 0.5
  dimension "d248" = 0.5
  dimension "d249" = 2.5
  dimension "d250" = 2.5
  dimension "d251" = 2.5
  dimension "d252" = 2.5
  constraint horizontal L12
  constraint vertical L13
  constraint horizontal L14
  constraint vertical L15
  constraint horizontal L17
  constraint vertical L18
  constraint horizontal L19
  constraint vertical L20
  measures "d245" distance of L11 L12
  measures "d246" distance of L9 L14
  measures "d247" distance of L15 L16
  measures "d248" distance of L10 L13
  measures "d249" distance of L20 L21
  measures "d250" distance of L6 L18
  measures "d251" distance of L7 L17
  measures "d252" distance of L5 L19
extrude "Extrude11" cut sketch "Sketch7" against normal blind 1.5 contours L4 L5 L6 L7 L21 | L8 L9 L10 L11 L16 | L12 L13 L14 L15 | L17 L18 L19 L20 bodies 6
sketch "Sketch8" plane through (65, 0, 0) normal (1, 0, 0) x (0, 0, -1)
  line L0 (-30, -65) -> (1.5, -65)
  line L1 (1.5, -65) -> (1.5, 65)
  line L2 (1.5, 65) -> (-30, 65)
  line L3 (-30, 65) -> (-30, -65)
  circle A0 centre (-14.25, 15) radius 1.75
  circle A1 centre (-14.25, -10) radius 1.75
  circle A2 centre (-14.25, -25) radius 1.75
  circle A3 centre (-14.25, -50) radius 1.75
  line L4 (-8.75, -27.85) -> (-8.75, -47.15)
  line L5 (-8.75, -47.15) -> (-19.75, -47.15)
  line L6 (-19.75, -47.15) -> (-19.75, -27.85)
  line L7 (-19.75, -27.85) -> (-8.75, -27.85)
  line L8 (-8.75, 12.15) -> (-8.75, -7.15)
  line L9 (-8.75, -7.15) -> (-19.75, -7.15)
  line L10 (-19.75, -7.15) -> (-19.75, 12.15)
  line L11 (-19.75, 12.15) -> (-8.75, 12.15)
extrude "Extrude12" cut sketch "Sketch8" against normal blind 1.5 contours A0 | A1 | A2 | A3 | L4 L5 L6 L7 | L8 L9 L10 L11 bodies 6
extrude "Extrude13" add sketch "Sketch6" against normal blind 4 contours A4 A9 | A5 A12 | A6 A13 | A7 A10 | A11 bodies 6
fillet "Fillet1'" radius 3 8 edges at (-65, -65, 14.25) (65, -65, 14.25) (65, 65, 14.25) (-65, 65, 14.25) (-65, -65, 53.6) (65, -65, 53.6) (65, 65, 53.6) (-65, 65, 53.6) on bodies 6 7
sketch "Sketch9" plane through (0, 0, 30) normal (0, 0, 1) x (1, 0, 0)
  circle A0 centre (-60.25, -60.25) radius 1.75
  circle A1 centre (-60.25, 60.25) radius 1.75
  circle A2 centre (60.25, -60.25) radius 1.75
  circle A3 centre (60.25, 60.25) radius 1.75
  line L0 (56.7859, -63.5) -> (-56.7859, -63.5)
  arc A4 (-56.7859, -63.5) -> (-63.5, -56.7859) centre (-60.25, -60.25) ccw
  line L1 (-63.5, -56.7859) -> (-63.5, 56.7859)
  arc A5 (-63.5, 56.7859) -> (-56.7859, 63.5) centre (-60.25, 60.25) ccw
  line L2 (-56.7859, 63.5) -> (56.7859, 63.5)
  arc A6 (56.7859, 63.5) -> (63.5, 56.7859) centre (60.25, 60.25) ccw
  line L3 (63.5, 56.7859) -> (63.5, -56.7859)
  arc A7 (63.5, -56.7859) -> (56.7859, -63.5) centre (60.25, -60.25) ccw
  arc A8 (-62, 65) -> (-65, 62) centre (-62, 62) ccw
  line L4 (-65, 62) -> (-65, -62)
  arc A9 (-65, -62) -> (-62, -65) centre (-62, -62) ccw
  line L5 (-62, -65) -> (62, -65)
  arc A10 (62, -65) -> (65, -62) centre (62, -62) ccw
  line L6 (65, -62) -> (65, 62)
  arc A11 (65, 62) -> (62, 65) centre (62, 62) ccw
  line L7 (62, 65) -> (-62, 65)
  line L8 (62, 64.2) -> (-62, 64.2)
  arc A12 (-62, 64.2) -> (-64.2, 62) centre (-62, 62) ccw
  line L9 (-64.2, 62) -> (-64.2, -62)
  arc A13 (-64.2, -62) -> (-62, -64.2) centre (-62, -62) ccw
  line L10 (-62, -64.2) -> (62, -64.2)
  arc A14 (62, -64.2) -> (64.2, -62) centre (62, -62) ccw
  line L11 (64.2, -62) -> (64.2, 62)
  arc A15 (64.2, 62) -> (62, 64.2) centre (62, 62) ccw
  arc A16 (-62, 64.3) -> (-64.3, 62) centre (-62, 62) ccw
  line L12 (-64.3, 62) -> (-64.3, -62)
  arc A17 (-64.3, -62) -> (-62, -64.3) centre (-62, -62) ccw
  line L13 (-62, -64.3) -> (62, -64.3)
  arc A18 (62, -64.3) -> (64.3, -62) centre (62, -62) ccw
  line L14 (64.3, -62) -> (64.3, 62)
  arc A19 (64.3, 62) -> (62, 64.3) centre (62, 62) ccw
  line L15 (62, 64.3) -> (-62, 64.3)
  line L16 (62, 63.5) -> (-62, 63.5)
  arc A20 (-62, 63.5) -> (-63.5, 62) centre (-62, 62) ccw
  line L17 (-63.5, 62) -> (-63.5, -62)
  arc A21 (-63.5, -62) -> (-62, -63.5) centre (-62, -62) ccw
  line L18 (-62, -63.5) -> (62, -63.5)
  arc A22 (62, -63.5) -> (63.5, -62) centre (62, -62) ccw
  line L19 (63.5, -62) -> (63.5, 62)
  arc A23 (63.5, 62) -> (62, 63.5) centre (62, 62) ccw
  dimension "d269" = -0.8
  dimension "d270" = -0.7
  dimension "d271" = -1.5
extrude "Extrude14" cut sketch "Sketch9" against normal blind 0.8 contours A8 L4 A9 L5 A10 L6 A11 L7 | A16 L12 A17 L13 A18 L14 A19 L15 bodies 6
extrude "Extrude15" cut sketch "Sketch9" along normal blind 0.8 contours A0 | A1 | A2 | A3 | A7 L18 A22 L19 | A4 L17 A21 L18 | A6 L16 L19 A23 | A5 L16 A20 L17 | L8 A12 L9 A13 L10 A14 L11 A15 | A16 L12 A17 L13 A18 L14 A19 L15 bodies 7
extrude "Extrude16" cut 1 faces at (2.4879, 9.8385, 30.1) along direction (0, 0, 1) blind 0.8 on bodies 7 bodies 7
sketch "Sketch10" plane through (63.5, 0, 0) normal (-1, 0, 0) x (0, 0, 1)
  circle A0 centre (14.25, -25) radius 1.75
  line L0 (19.75, -7.15) -> (8.75, -7.15)
  line L1 (8.75, -7.15) -> (8.75, 12.15)
  line L2 (8.75, 12.15) -> (19.75, 12.15)
  line L3 (19.75, 12.15) -> (19.75, -7.15)
  line L4 (19.75, -47.15) -> (8.75, -47.15)
  line L5 (8.75, -47.15) -> (8.75, -27.85)
  line L6 (8.75, -27.85) -> (19.75, -27.85)
  line L7 (19.75, -27.85) -> (19.75, -47.15)
  circle A1 centre (14.25, -10) radius 1.75
  circle A2 centre (14.25, 15) radius 1.75
  circle A3 centre (14.25, -50) radius 1.75
  line L8 (0, -56.7859) -> (30, -56.7859)
  line L9 (30, -56.7859) -> (30, 56.7859)
  line L10 (30, 56.7859) -> (0, 56.7859)
  line L11 (0, 56.7859) -> (0, -56.7859)
  line L12 (5.75, 19) -> (22.75, 19)
  line L13 (22.75, 19) -> (22.75, -54)
  line L14 (22.75, -54) -> (5.75, -54)
  line L15 (5.75, -54) -> (5.75, 19)
  circle A4 centre (14.25, 15) radius 1.75
  dimension "d278" = 3
  dimension "d279" = 3
  constraint horizontal L12
  constraint vertical L13
  constraint horizontal L14
  constraint vertical L15
  measures "d278" distance of L1 L15
  measures "d279" distance of L3 L13
extrude "Extrude17" add sketch "Sketch10" along normal blind 1 contours L12 L13 L14 L15 bodies 6
chamfer "Chamfer1" distance 1 angle 45 1 edges at (63.5, -17.5, 5.75) on bodies 6
chamfer "Chamfer2" distance 1 angle 45 21 edges at (0, -65, 77.1) (-64.1213, -64.1213, 77.1) (-65, 0, 77.1) (-64.1213, 64.1213, 77.1) (0, 65, 77.1) (64.1213, 64.1213, 77.1) (65, 0, 77.1) (64.1213, -64.1213, 77.1) (0, -63.5, 75.6) (-57.9519, -57.9519, 75.6) (-49.297, -59.7098, 75.6) (43.703, -59.7098, 75.6) (43.703, -4.4598, 75.6) (-49.297, -4.4598, 75.6) (-3.0301, 8.8248, 75.6) (57.9519, 57.9519, 75.6) (0, 63.5, 75.6) (-57.9519, 57.9519, 75.6) (63.5, 0, 75.6) (57.9519, -57.9519, 75.6) (-63.5, 0, 75.6) on bodies 7
chamfer "Chamfer3" distance 1 angle 45 29 edges at (64.1213, -64.1213, -1.5) (0, -65, -1.5) (-64.1213, -64.1213, -1.5) (-65, 0, -1.5) (-64.1213, 64.1213, -1.5) (0, 65, -1.5) (64.1213, 64.1213, -1.5) (65, 0, -1.5) (0, 63.5, 0) (38.4699, 60.6753, 0) (15.4699, 60.6753, 0) (-21.5301, 60.6753, 0) (-44.5301, 60.6753, 0) (-44.5301, 21.6753, 0) (-21.5301, 21.6753, 0) (-4.4286, 11.7177, 0) (38.4699, 21.6753, 0) (56.8912, 56.8912, 0) (63.5, 0, 0) (-0.2301, -14.9747, 0) (-51.0301, 0.2253, 0) (-56.8912, 56.8912, 0) (15.4699, 21.6753, 0) (-63.5, 0, 0) (-52.3301, -47.9747, 0) (-0.2301, -42.8747, 0) (56.8912, -56.8912, 0) (0, -63.5, 0) (-56.8912, -56.8912, 0) on bodies 6
component "LCD-20x4" placed x (-1, 0, 0) y (0, 0, -1) z (0, -1, 0) at (0, -31, 67.5)
component "db9" placed x (0, -1, 0) y (0, 0, -1) z (1, 0, 0) at (66, -37.5, 14.25)
component "ArduinoWithCNCshield" placed x (1, 0, 0) y (0, 1, 0) z (0, 0, 1) at (-63.3, -51.65, 10.2)
component "BananaSockets" placed x (1, 0, 0) y (0, 1, 0) z (0, 0, 1) at (0, 0, 0)
component "RelayBoards" placed x (1, 0, 0) y (0, 1, 0) z (0, 0, 1) at (0, 0, 0)
component "db9" placed x (0, -1, 0) y (0, 0, -1) z (1, 0, 0) at (66, 2.5, 14.25)
component "BananaSocket" placed x (1, 0, 0) y (0, 1, 0) z (0, 0, 1) at (23.25, 18, 77.1) in component "BananaSockets"
component "BananaSocket" placed x (1, 0, 0) y (0, 1, 0) z (0, 0, 1) at (47, 48, 77.1) in component "BananaSockets"
component "BananaSocket" placed x (1, 0, 0) y (0, 1, 0) z (0, 0, 1) at (11.375, 33, 77.1) in component "BananaSockets"
component "BananaSocket" placed x (1, 0, 0) y (0, 1, 0) z (0, 0, 1) at (35.125, 33, 77.1) in component "BananaSockets"
component "BananaSocket" placed x (1, 0, 0) y (0, 1, 0) z (0, 0, 1) at (-24.25, 48, 77.1) in component "BananaSockets"
component "BananaSocket" placed x (1, 0, 0) y (0, 1, 0) z (0, 0, 1) at (23.25, 48, 77.1) in component "BananaSockets"
component "BananaSocket" placed x (1, 0, 0) y (0, 1, 0) z (0, 0, 1) at (-48, 18, 77.1) in component "BananaSockets"
component "BananaSocket" placed x (1, 0, 0) y (0, 1, 0) z (0, 0, 1) at (-48, 48, 77.1) in component "BananaSockets"
component "BananaSocket" placed x (1, 0, 0) y (0, 1, 0) z (0, 0, 1) at (-24.25, 18, 77.1) in component "BananaSockets"
component "BananaSocket" placed x (1, 0, 0) y (0, 1, 0) z (0, 0, 1) at (47, 18, 77.1) in component "BananaSockets"
component "RelayBoard" placed x (0, 1, 0) y (-1, 0, 0) z (0, 0, 1) at (-30, 40, 10) in component "RelayBoards"
component "RelayBoard" placed x (0, 1, 0) y (-1, 0, 0) z (0, 0, 1) at (30, 40, 10) in component "RelayBoards"
equation "d25 = d24 / 2"
equation "d67 = d66 / 2"
equation "d153 = d152 / 2"
equation "d201 = d200"
equation "d202 = d200"
equation "d203 = d200"
equation "d227 = d226"
equation "d228 = d226"
equation "d229 = d226"
equation "d230 = d226"
equation "d231 = d226"
equation "d232 = d226"
equation "d233 = d226"
equation "d234 = d226"
equation "d235 = d226"
equation "d236 = d226"
equation "d237 = d226"
equation "d239 = d238"
equation "d240 = d238"
equation "d241 = d238"
equation "d250 = d249"
equation "d251 = d249"
equation "d252 = d249"
named bodies: "ArdCtrlBottom", "ArdCtrlTop"
